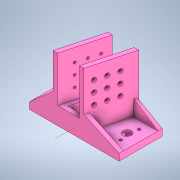
# Autodesk Inventor part: bracketForGarageUpperHalf
Saved by Autodesk Inventor 2022.1 (Build 261234020, 234B)
## iProperties
Created: 2021-10-20
Part Number: bracketForGarageUpperHalf
Material: PC/ABS Plastic
Document SubType Name: Modeling
Designer: robst
Density: 0.357273 g/cm^3
Appearance: Pink
Author: robst
Autodesk Inventor part; units mm, degrees
note: some values were not read from the file. Chosen so that the rebuilt part matches the saved one: direction of "HoleForLeftSideOf2x4"; direction of "HolesForRightSideOf2x4".
ref_plane "YZ Plane" through (0, 0, 0) normal (1, 0, 0) x (0, 1, 0)
ref_plane "XZ Plane" through (0, 0, 0) normal (0, 1, 0) x (-1, 0, 0)
sketch "Sketch8" plane through (0, 0, 0) normal (0, 1, 0) x (-1, 0, 0)
  line L0 (83, 40) -> (-83, 40)
  line L1 (-83, 40) -> (-83, -40)
  line L2 (-83, -40) -> (83, -40)
  line L3 (83, -40) -> (83, 40)
  line L4 (83, 40) -> (-83, -40) construction
  line L5 (-83, 40) -> (83, -40) construction
  point P0 (0, 0)
  dimension "d28" = 80
  dimension "d29" = 166
  constraints: 12 end point, 2 midpoint, 2 parallel, 1 horizontal, 1 perpendicular
  measures "d28" distance of L2.end L0.start
  measures "d29" distance between parallel lines of L1 L3
extrude "Extrusion8" add sketch "Sketch8" against normal blind 8
sketch "Sketch9" plane through (0, -8, 0) normal (0, -1, 0) x (1, 0, 0)
  line L0 (83, 40) -> (-83, 40) projected
  line L1 (-83, -40) -> (83, -40) projected
  line L2 (-83, 40) -> (-75, 40)
  line L3 (-75, 40) -> (-75, -40)
  line L4 (-75, -40) -> (-83, -40)
  line L5 (-83, -40) -> (-83, 40)
  line L6 (83, -40) -> (83, 40) projected
  line L7 (83, -40) -> (75, -40)
  line L8 (75, -40) -> (75, 40)
  line L9 (75, 40) -> (83, 40)
  line L10 (83, 40) -> (83, -40)
  point P0 (0, 0)
  point P1 (75, 40)
  point P2 (75, -40)
  dimension "d32" = 8
  dimension "d33" = 8
  constraints: 16 end point, 4 parallel, 2 horizontal, 2 perpendicular, 2 point on line
  measures "d32" distance between parallel lines of L3 L5
  measures "d33" distance between parallel lines of L6 L8
extrude "armsForCameraCase" add sketch "Sketch9" along normal blind 140 contours L6 L1 L8 L0 | L3 L1 L5 L0
sketch "Sketch10" plane through (-75, -8, 40) normal (1, 0, 0) x (0, 0, -1)
  line L0 (0, 0) -> (80, 0)
  line L1 (80, 0) -> (80, -140)
  line L2 (80, -140) -> (0, -140)
  line L3 (0, 0) -> (0, -140)
  line L4 (0, 0) -> (80, -29.117619)
  line L5 (80, -29.117619) -> (80, 0)
  line L6 (80, 0) -> (0, 0)
  point P0 (40, 8)
  point P1 (40, -14.558809)
  dimension "d48" = 20
  constraints: 6 end point, 2 collinear, 1 midpoint, 1 point on line
  measures "d48" angle of L4 L0
extrude "Extrusion10" add sketch "Sketch10" along normal up to surface (150 mm away) contours L0 L1 L4
sketch "Sketch11" plane through (0, 0, 0) normal (0, 1, 0) x (1, 0, 0)
  line L0 (83, 40) -> (-83, 40)
  line L1 (-83, -40) -> (83, -40)
  line L2 (-83, 40) -> (-83, -40)
  line L3 (83, -40) -> (83, 40)
  line L4 (-31.037968, -40) -> (-9.602032, 40)
  line L5 (-9.602032, 40) -> (-17.884242, 40)
  line L6 (-75, 40) -> (75, 40)
  line L7 (-17.884242, 40) -> (-39.320177, -40)
  line L8 (-39.320177, -40) -> (-31.037968, -40)
  line L9 (-31.037968, -40) -> (-31.037968, 40) construction
  line L10 (0, -40) -> (0, 40) construction
  line L11 (9.602032, -40) -> (31.037968, 40)
  line L12 (31.037968, 40) -> (39.320177, 40)
  line L13 (39.320177, 40) -> (17.884242, -40)
  line L14 (17.884242, -40) -> (9.602032, -40)
  point P0 (0, 0)
  point P1 (0, -40)
  point P2 (0, -40)
  point P3 (-20.32, 0)
  point P4 (0, 0)
  point P5 (20.32, 0)
  point P6 (39.320177, 40)
  point P7 (31.037968, 40)
  point P8 (-17.884242, 40)
  dimension "d39" = -15
  dimension "d40" = 8
  dimension "d42" = 8
  dimension "d44" = 20.32
  dimension "d45" = 20.32
  constraints: 20 end point, 5 point on line, 4 midpoint, 3 parallel, 2 horizontal, 1 perpendicular, 8 other
  measures "d39" angle of L4 L9
  measures "d40" distance between parallel lines of L7 L4
  measures "d42" distance between parallel lines of L13 L11
  measures "d44" distance of point (-20.32, 0) point (0, 0)
  measures "d45" distance of point (20.32, 0) point (0, 0)
extrude "Extrusion11" add sketch "Sketch11" along normal blind 104.1375 contours L13 L1 L11 L0 | L4 L1 L7 L0
sketch "Sketch12" plane through (0, 0, 0) normal (0, 1, 0) x (1, 0, 0)
  line L0 (31.037968, 40) -> (-9.602032, 40)
  line L1 (31.037968, 40) -> (9.602032, -40)
  line L2 (-31.037968, -40) -> (9.602032, -40)
  line L3 (-31.037968, -40) -> (-9.602032, 40)
  line L4 (-9.602032, 40) -> (31.037968, 40)
  line L5 (31.037968, 40) -> (9.602032, -40)
  line L6 (9.602032, -40) -> (-31.037968, -40)
  line L7 (-9.602032, 40) -> (-31.037968, -40)
  line L8 (-31.037968, -40) -> (-9.602032, 40)
  point P0 (0, 0)
  constraints: 8 end point, 3 equal length
extrude "Extrusion12" add sketch "Sketch12" along normal blind 20
sketch "Sketch13" plane through (-83, 0, -40) normal (-1, 0, 0) x (0, 0, 1)
  line L0 (0, -37.117619) -> (80, -8)
  line L1 (80, 0) -> (80, -148)
  line L2 (80, -148) -> (0, -148)
  line L3 (0, 0) -> (0, -148)
  line L4 (80, -148) -> (0, -148) construction
  line L5 (40, -148) -> (40, -22.558809) construction
  line L6 (80, -8) -> (0, -37.117619) construction
  line L7 (0, -132.893618) -> (80, -103.776) construction
  line L8 (80, -8) -> (80, -148) construction
  point P0 (40, 0)
  point P1 (40, -118.334809)
  point P2 (20, -125.614214)
  point P3 (60, -111.055404)
  dimension "centerForTwoHoles" = 21.28356
  dimension "d51" = 90
  dimension "diagonalLine" = 85.13422
  dimension "d62" = 21.28356
  dimension "d63" = 21.28356
  constraints: 4 end point, 4 point on line, 3 midpoint, 1 parallel
  measures "d51" distance between parallel lines of L7 L0
  measures "diagonalLine" distance of L7.start L7.end
  measures "d62" distance of point (20, -125.614) L7.start
  measures "d63" distance of point (60, -111.055) L7.end
hole "Hole1" at (-83, -118.334809, 0) at (-83, -125.614214, -20) at (-83, -111.055404, 20) direction (1, 0, 0) diameter 6.7564 end through all clearance for "Hex Machine Screw" size "1/4" standard "Ansi Unified Screw Threads"
sketch "Sketch14" plane through (-83, 0, -40) normal (-1, 0, 0) x (0, 0, 1)
  line L0 (80, 0) -> (80, -148)
  line L1 (80, -148) -> (0, -148)
  line L2 (0, 0) -> (0, -148)
  line L3 (0, -37.117619) -> (80, -8)
  line L4 (0, -37.117619) -> (0, -148)
  line L5 (0, -148) -> (80, -118.882381)
  line L6 (0, -148) -> (80, -148)
  line L7 (0, -148) -> (80, -148)
  line L8 (80, -148) -> (80, -118.882381)
  point P0 (40, 0)
  constraints: 6 end point, 2 collinear, 1 parallel, 1 point on line
extrude "Extrusion13" cut sketch "Sketch14" against normal through all contours L0 L1 L5
sketch "Sketch15" plane through (-39.320177, 0, 40) normal (-0.9659258, 0, -0.258819) x (-0.258819, 0, 0.9659258)
  line L0 (-82.822094, 104.1375) -> (0, 104.1375)
  line L1 (0, 0) -> (0, 104.1375)
  line L2 (-82.822094, 0) -> (-82.822094, 104.1375)
  line L3 (-2.143594, 20) -> (-84.965688, 20)
  line L4 (-82.822094, 40) -> (0, 40) construction
  line L5 (-67.822094, 40) -> (-67.822094, 104.1375) construction
  point P0 (-48.813844, 0)
  point P1 (-82.822094, 52.06875)
  point P2 (-47.822094, 40)
  point P3 (-27.822094, 40)
  point P4 (-67.822094, 60)
  point P5 (-47.822094, 60)
  point P6 (-27.822094, 60)
  point P7 (-67.822094, 80)
  point P8 (-47.822094, 80)
  point P9 (-27.822094, 80)
  dimension "d64" = 15
  dimension "d74" = 20
  dimension "d77" = 20
  dimension "d90" = 20
  constraints: 4 end point, 4 point on line, 2 perpendicular, 1 coincident, 1 horizontal, 1 midpoint, 1 vertical, 8 other
  measures "d64" distance from line of point (-82.822, 52.069) L5
  measures "d74" distance of point (-67.822, 40) point (-47.822, 40)
  measures "d77" distance of point (-67.822, 40) point (-67.822, 60)
  measures "d90" distance between parallel lines of L4 L3
hole "HoleForLeftSideOf2x4" at (-21.766527, 40, -25.511113) at (-26.942908, 40, -6.192596) at (-32.119289, 40, 13.12592) at (-26.942908, 60, -6.192596) at (-21.766527, 60, -25.511113) at (-32.119289, 60, 13.12592) at (-32.119289, 80, 13.12592) at (-26.942908, 80, -6.192596) at (-21.766527, 80, -25.511113) direction (0.9659258, 0, 0.258819) diameter 4.496 depth 8 countersink diameter 8.433 countersink angle 82 clearance for "Flat Head Machine Screw (82)" size "#8" standard "Ansi Unified Screw Threads"
sketch "Sketch16" plane through (39.320177, 0, -40) normal (0.9659258, 0, 0.258819) x (0.258819, 0, -0.9659258)
  line L0 (-82.822094, 104.1375) -> (0, 104.1375)
  line L1 (0, 0) -> (0, 104.1375)
  line L2 (-82.822094, 0) -> (-82.822094, 104.1375)
  line L3 (-82.822094, 0) -> (-65.968896, 0)
  line L4 (-2.143594, 20) -> (-84.965688, 20)
  line L5 (-82.822094, 40) -> (0, 40) construction
  line L6 (-67.822094, 40) -> (-67.822094, 104.1375) construction
  point P0 (-48.813844, 0)
  point P1 (-47.822094, 40)
  point P2 (-27.822094, 40)
  point P3 (-67.822094, 60)
  point P4 (-47.822094, 60)
  point P5 (-27.822094, 60)
  point P6 (-67.822094, 80)
  point P7 (-47.822094, 80)
  point P8 (-27.822094, 80)
  dimension "d80" = 20
  dimension "d81" = 15
  dimension "d84" = 20
  dimension "d87" = 20
  constraints: 4 end point, 4 point on line, 2 perpendicular, 1 coincident, 1 horizontal, 1 vertical, 8 other
  measures "d80" distance between parallel lines of L5 L4
  measures "d81" distance between parallel lines of L6 L2
  measures "d84" distance of point (-67.822, 40) point (-47.822, 40)
  measures "d87" distance of point (-67.822, 40) point (-67.822, 60)
hole "HolesForRightSideOf2x4" at (26.942908, 40, 6.192596) at (32.119289, 40, -13.12592) at (21.766527, 60, 25.511113) at (26.942908, 60, 6.192596) at (32.119289, 60, -13.12592) at (21.766527, 80, 25.511113) at (26.942908, 80, 6.192596) at (32.119289, 80, -13.12592) at (21.766527, 40, 25.511113) direction (-0.9659258, 0, -0.258819) diameter 4.496 depth 8 countersink diameter 8.433 countersink angle 82 clearance for "Flat Head Machine Screw (82)" size "#8" standard "Ansi Unified Screw Threads"
sketch "Sketch17" plane through (0, 20, 0) normal (0, 1, 0) x (1, 0, 0)
  line L0 (31.037968, 40) -> (9.602032, -40)
  line L1 (-31.037968, -40) -> (9.602032, -40)
  line L2 (-31.037968, -40) -> (-9.602032, 40)
  line L3 (31.037968, 40) -> (-9.602032, 40)
  line L4 (20.612165, 32) -> (3.463416, -32)
  line L5 (3.463416, -32) -> (-20.612165, -32)
  line L6 (-20.612165, -32) -> (-3.463416, 32)
  line L7 (-3.463416, 32) -> (20.612165, 32)
  point P0 (0, 0)
  point P1 (10.717968, 40)
  point P2 (-8.574374, -32)
  dimension "d98" = 8
  dimension "d99" = 8
  dimension "d101" = 8
  dimension "d102" = 8
  constraints: 8 end point, 4 parallel, 2 midpoint, 1 horizontal
  measures "d98" distance between parallel lines of L4 L0
  measures "d99" distance between parallel lines of L6 L2
  measures "d101" distance from line of point (10.718, 40) L7
  measures "d102" distance from line of point (-8.574, -32) L1
extrude "Extrusion14" cut sketch "Sketch17" against normal through all contours L4 L5 L6 L7
sketch "Sketch18" plane through (0, 0, 0) normal (0, 1, 0) x (1, 0, 0)
  line L0 (17.884242, -40) -> (83, -40)
  line L1 (17.884242, -40) -> (39.320177, 40)
  line L2 (83, 40) -> (39.320177, 40)
  line L3 (83, -40) -> (83, 40)
  line L4 (67, -32) -> (67, 32)
  line L5 (67, 32) -> (45.458793, 32)
  line L6 (45.458793, 32) -> (28.310045, -32)
  line L7 (28.310045, -32) -> (67, -32)
  line L8 (39.320177, 40) -> (17.884242, -40)
  line L9 (17.884242, -40) -> (83, -40)
  line L10 (83, -40) -> (83, 40)
  line L11 (83, 40) -> (39.320177, 40)
  point P0 (0, 0)
  dimension "d105" = 8
  dimension "d107" = 8
  dimension "d108" = 16
  dimension "d109" = 8
  constraints: 8 end point, 4 parallel, 1 perpendicular
  measures "d105" distance between parallel lines of L7 L0
  measures "d107" distance between parallel lines of L1 L6
  measures "d108" distance between parallel lines of L3 L4
  measures "d109" distance between parallel lines of L5 L2
extrude "Extrusion15" cut sketch "Sketch18" against normal through all contours L7 L6 L5 L4
sketch "Sketch19" plane through (0, 0, 0) normal (0, 1, 0) x (1, 0, 0)
  line L0 (-17.884242, 40) -> (-39.320177, -40)
  line L1 (-83, -40) -> (-39.320177, -40)
  line L2 (-83, 40) -> (-83, -40)
  line L3 (-17.884242, 40) -> (-83, 40)
  line L4 (-28.310045, 32) -> (-45.458793, -32)
  line L5 (-45.458793, -32) -> (-67, -32)
  line L6 (-67, -32) -> (-67, 32)
  line L7 (-67, 32) -> (-28.310045, 32)
  point P0 (0, 0)
  point P1 (-61.160089, -40)
  dimension "d112" = 8
  dimension "d113" = 16
  dimension "d114" = 8
  dimension "d115" = 8
  constraints: 8 end point, 4 parallel, 1 horizontal, 1 midpoint
  measures "d112" distance between parallel lines of L0 L4
  measures "d113" distance between parallel lines of L6 L2
  measures "d114" distance from line of point (-61.16, -40) L5
  measures "d115" distance between parallel lines of L3 L7
extrude "Extrusion16" cut sketch "Sketch19" against normal through all contours L4 L5 L6 L7
sketch "Sketch27" plane through (-75, -8, 40) normal (0, 0, 1) x (1, 0, 0)
  line L0 (92.884242, 8) -> (158, 8)
  line L1 (92.884242, 8) -> (92.884242, 112.1375)
  line L2 (158, 8) -> (158, -110.882381)
  line L3 (92.884242, 38) -> (158, 8)
  line L4 (158, 8) -> (92.884242, 8)
  line L5 (92.884242, 8) -> (92.884242, 38)
  point P0 (75, 8)
  dimension "d152" = 30
  constraints: 6 end point, 2 collinear, 1 point on line
  measures "d152" distance of L0.start L3.start
sketch "Sketch28" plane through (67, 0, 32) normal (0, 0, -1) x (-1, 0, 0)
  line L0 (-16, 0) -> (47.939383, 0)
  line L1 (49.115758, 0) -> (49.115758, 104.1375)
  line L2 (47.939383, 0) -> (47.939383, 30)
  line L3 (47.939383, 30) -> (-16, 0)
  point P0 (67, 0)
  dimension "d153" = 30
  constraints: 6 end point, 1 parallel, 1 perpendicular
  measures "d153" distance of L0.end L2.end
loft "Loft5" add profiles "Sketch27", "Sketch28"
sketch "Sketch29" plane through (75, -37.117619, -40) normal (0, 0, -1) x (-1, 0, 0)
  line L0 (-8, 37.117619) -> (44, 37.117619)
  line L1 (44, 37.117619) -> (44, 242.855119)
  line L2 (-8, 37.117619) -> (-8, -81.764763)
  line L3 (-8, 37.117619) -> (44, 37.117619)
  line L4 (44, 37.117619) -> (44, 67.117619)
  line L5 (44, 67.117619) -> (-8, 37.117619)
  point P0 (75, 37.117619)
  dimension "d158" = 30
  dimension "d217" = 52
  constraints: 10 end point, 1 collinear, 1 point on line
  measures "d158" distance of L4.end L0.end
  measures "d217" distance from line of L1 L0.start
sketch "Sketch30 outline for Loft6" plane through (45.458793, 0, -32) normal (0, 0, 1) x (1, 0, 0)
  line L0 (-6.138616, 28.823162) -> (-14.458793, 0)
  line L1 (37.541207, 0) -> (-6.138616, 28.823162)
  line L2 (-14.458793, 0) -> (37.541207, 0)
loft "Loft6" add profiles "Sketch29", "Sketch30 outline for Loft6"
sketch "Sketch31" plane through (-75, -8, 40) normal (0, 0, 1) x (1, 0, 0)
  line L0 (-8, 8) -> (35.679823, 8)
  line L1 (35.679823, 8) -> (35.679823, 112.1375)
  line L2 (57.115758, 8) -> (-8, 8)
  line L3 (-8, 8) -> (35.679823, 8)
  line L4 (35.679823, 8) -> (35.679823, 47)
  line L5 (35.679823, 47) -> (-8, 8)
  point P0 (75, 8)
  dimension "d164" = 39
  constraints: 6 end point, 1 horizontal, 1 point on line
  measures "d164" distance of L4.end L0.end
sketch "Sketch32" plane through (-45.458793, 0, 32) normal (0, 0, -1) x (-1, 0, 0)
  line L0 (37.541207, 0) -> (-6.138616, 0)
  line L1 (37.541207, 0) -> (-8.745784, 0)
  line L2 (-8.745784, 0) -> (-8.745784, 30)
  line L3 (-8.745784, 30) -> (37.541207, 0)
  point P0 (-45.458793, 0)
  dimension "d165" = 30
  constraints: 6 end point, 1 horizontal, 1 perpendicular
  measures "d165" distance of L1.end L2.end
sketch "Sketch31 outline for Loft7" plane through (-75, -8, 40) normal (0, 0, 1) x (1, 0, 0)
  line L0 (35.679823, 47) -> (-8, 8)
  line L1 (35.679823, 8) -> (35.679823, 47)
  line L2 (-8, 8) -> (35.679823, 8)
sketch "Sketch32 outline for Loft7" plane through (-45.458793, 0, 32) normal (0, 0, -1) x (-1, 0, 0)
  line L0 (37.541207, 0) -> (-8.745784, 0)
  line L1 (-8.745784, 0) -> (-8.745784, 30)
  line L2 (-8.745784, 30) -> (37.541207, 0)
loft "Loft7" add profiles "Sketch31 outline for Loft7", "Sketch32 outline for Loft7"
sketch "Sketch33" plane through (75, -37.117619, -40) normal (0, 0, -1) x (-1, 0, 0)
  line L0 (92.884242, 37.117619) -> (158, 37.117619)
  line L1 (92.884242, 37.117619) -> (92.884242, 141.255119)
  line L2 (112.176584, 37.117619) -> (92.884242, 37.117619)
  line L3 (92.884242, 37.117619) -> (158, 37.117619)
  line L4 (158, 37.117619) -> (92.884242, 67.117619)
  line L5 (92.884242, 67.117619) -> (92.884242, 37.117619)
  point P0 (75, 37.117619)
  dimension "d171" = 30
  constraints: 6 end point, 2 collinear, 1 point on line
  measures "d171" distance of L4.end L0.start
sketch "Sketch34" plane through (-67, 0, -32) normal (0, 0, 1) x (1, 0, 0)
  line L0 (49.115758, 0) -> (-16, 0)
  line L1 (49.115758, 0) -> (49.115758, 104.1375)
  line L2 (-16, 0) -> (50.026246, 0)
  line L3 (29.823416, 0) -> (49.115758, 0)
  line L4 (50.026246, 0) -> (50.026246, 30)
  line L5 (50.026246, 30) -> (-16, 0)
  point P0 (67, 0)
  dimension "d170" = 30
  constraints: 6 end point, 1 point on line, 1 vertical
  measures "d170" distance of L2.end L4.end
loft "Loft8" add profiles "Sketch33", "Sketch34"
split "Split3" plane through (0, 0, 0) removes the side toward (0, -1, 0)
sketch "Sketch40" plane through (83, 0, 32) normal (0, -1, 0) x (1, 0, 0)
  line L0 (-166, 8) -> (0, 8) projected
  line L1 (0, -72) -> (-166, -72) projected
  line L2 (0, 8) -> (0, 0) projected
  line L3 (0, -64) -> (0, -72) projected
  line L4 (-166, -72) -> (-166, -64) projected
  line L5 (-166, 0) -> (-166, 8) projected
  line L6 (0, -72) -> (-166, -72) projected
  line L7 (-166, -72) -> (0, -72)
  line L8 (0, -72) -> (0, 8)
  line L9 (0, 8) -> (-166, 8)
  line L10 (-166, 8) -> (-166, -72)
  line L11 (-166, -72) -> (0, 8) construction
  line L12 (0, -72) -> (-166, 8) construction
  point P0 (-83, -32)
  point P1 (-43.679823, -72)
  point P2 (-166, -64)
  constraints: 12 end point, 2 midpoint, 2 parallel, 1 horizontal, 1 perpendicular
extrude "ExtrusionForMatingToLowerHalf" add sketch "Sketch40" along normal blind 12.5
sketch "Sketch42" plane through (83, 0, 32) normal (0, 1, 0) x (1, 0, 0)
  line L0 (-166, 0) -> (-166, 64) projected
  line L1 (0, 64) -> (0, 0) projected
  point P0 (-146, 49)
  point P1 (-20, 49)
  point P2 (-20, 15)
  point P3 (-146, 15)
  dimension "d202" = 20
  dimension "d203" = 20
  dimension "d204" = 20
  dimension "d205" = 20
  dimension "d218" = 126
  dimension "d219" = 34
  measures "d202" distance from line of L0 point (-146, 49)
  measures "d203" distance from line of L0 point (-146, 15)
  measures "d204" distance from line of L1 point (-20, 49)
  measures "d205" distance from line of point (-20, 15) L1
  measures "d218" distance of point (-20, 49) point (-146, 49)
  measures "d219" distance of point (-146, 15) point (-146, 49)
hole "Hole5" at (-63, 0, -17) at (63, 0, -17) at (63, 0, 17) at (-63, 0, 17) direction (0, -1, 0) diameter 5.1054 end through all
ref_plane "Work Plane3" through (-33.5, 0, -32) normal (0, -0.9396926, 0.3420201) x (1, 0, 0)
sketch "SketchForHoleToSupportCase" plane through (-33.5, 0, -32) normal (0, -0.9396926, 0.3420201) x (1, 0, 0)
  line L0 (-49.5, 60.140328) -> (-49.5, 0)
  line L1 (116.5, 0) -> (116.5, 60.140328)
  line L2 (116.5, 60.140328) -> (53.527835, 60.140328)
  line L3 (-49.5, 60.140328) -> (-3.676584, 60.140328)
  line L4 (116.5, 30.140328) -> (-49.5, 30.140328) construction
  circle A0 centre (91.5, 30.140328) radius 2.5527
  circle A1 centre (-24.5, 30.140328) radius 2.5527
  circle A2 centre (91.5, 30.140328) radius 7.5
  circle A3 centre (-24.5, 30.140328) radius 7.5
  point P0 (33.5, 30.070164)
  dimension "d208" = 30
  dimension "d209" = 5.1054
  dimension "d210" = 25
  dimension "d211" = 25
  dimension "d214" = 15
  constraints: 4 centre point, 4 point on line, 2 coincident, 2 end point, 2 equal radius, 1 perpendicular
  measures "d208" distance between parallel lines of L4 L2
  measures "d209" diameter of A0
  measures "d210" distance from line of A0.centre L1
  measures "d211" distance from line of A1.centre L0
  measures "d214" diameter of A2
extrude "ExtrusionFor10Screw" cut sketch "SketchForHoleToSupportCase" along normal up to surface contours A0 | A1 surface through (0, -12.5, 0) normal (0, -1, 0)
extrude "ExtrusionForWasher" cut sketch "SketchForHoleToSupportCase" along normal blind 14 contours A0 | A1 | A2 | A3
sketch "Sketch30" plane through (45.458793, 0, -32) normal (0, 0, 1) x (1, 0, 0)
  line L0 (-14.458793, 0) -> (-14.458793, 205.7375)
  line L1 (37.541207, 0) -> (-14.458793, 0)
  line L2 (-6.138616, 0) -> (-6.138616, 205.7375)
  line L3 (-14.458793, 0) -> (37.541207, 0)
  line L4 (37.541207, 0) -> (-6.138616, 28.823162)
  line L5 (-6.138616, 28.823162) -> (-6.138616, 0)
  point P0 (-45.458793, 0)
  dimension "d159" = 30
  constraints: 6 end point, 1 horizontal, 1 parallel, 2 other
  measures "d159" distance of L4.end L0.start
equation "\"d28\" = widthOfBracket"
equation "\"d30\" = wallThickness"
equation "\"d32\" = wallThickness"
equation "\"d33\" = wallThickness"
equation "\"d34\" = bracketLength"
equation "\"d48\" = elevation"
equation "\"d39\" = azimuth"
equation "\"d40\" = wallThickness"
equation "\"d42\" = wallThickness"
equation "\"d44\" = 0.5 * twoByFourWidth"
equation "\"d45\" = 0.5 * twoByFourWidth"
equation "\"d46\" = twoByFourDepth + baseBelowTwoByFour"
equation "\"d49\" = baseBelowTwoByFour"
equation "\"centerForTwoHoles\" = 0.25 * diagonalLine"
equation "\"d62\" = centerForTwoHoles"
equation "\"d63\" = centerForTwoHoles"
equation "\"d98\" = wallThickness"
equation "\"d99\" = wallThickness"
equation "\"d101\" = wallThickness"
equation "\"d102\" = wallThickness"
equation "\"d105\" = wallThickness"
equation "\"d107\" = wallThickness"
equation "\"d108\" = 2 * wallThickness"
equation "\"d109\" = wallThickness"
equation "\"d112\" = wallThickness"
equation "\"d113\" = 2 * wallThickness"
equation "\"d114\" = wallThickness"
equation "\"d115\" = wallThickness"
equation "\"d191\" = depthOfExtrusionForMatingToLowerHalf"
equation "\"d215\" = depthForWasherForMatingToCase"
equation "\"wallThickness\" = 8"
equation "\"widthOfBracket\" = 80"
equation "\"twoByFourWidth\" = 40.64"
equation "\"twoByFourDepth\" = 84.1375"
equation "\"azimuth\" = -15deg"
equation "\"elevation\" = 20deg"
equation "\"baseBelowTwoByFour\" = 20"
equation "\"bracketLength\" = 140"
equation "\"depthOfExtrusionForMatingToLowerHalf\" = 12.5"
equation "\"depthForWasherForMatingToCase\" = 14"
body "Solid2"
